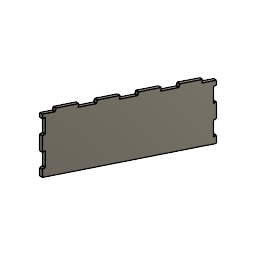
Deksel Volledig (Autodesk Fusion 360 archive; units mm, degrees)
design "de korte muur"
part number: 2026-02-05-13-28-29-515
part number: 2026-02-05-14-14-12-831
Autodesk Fusion 360 part; units mm, degrees
sketch "Sketch1" plane through (0, 0, 0) normal (0, 0, 1) x (1, 0, 0)
  line L0 (-114.5247, 50) -> (865.4753, 50)
  line L1 (865.4753, 50) -> (865.4753, -330)
  line L2 (865.4753, -330) -> (-114.5247, -330)
  line L3 (-114.5247, -330) -> (-114.5247, 50)
  line L4 (130.4753, 50) -> (130.4753, -330) construction
  line L5 (375.4753, -330) -> (375.4753, 50) construction
  line L6 (620.4753, 50) -> (620.4753, -330) construction
  line L7 (-39.5247, 0) -> (55.4753, 0)
  line L8 (80.4753, -25) -> (80.4753, -255)
  line L9 (55.4753, -280) -> (-39.5247, -280)
  line L10 (-64.5247, -255) -> (-64.5247, -25)
  line L11 (695.4753, 0) -> (790.4753, 0)
  line L12 (815.4753, -25) -> (815.4753, -255)
  line L13 (790.4753, -280) -> (695.4753, -280)
  line L14 (670.4753, -255) -> (670.4753, -25)
  arc A0 (-39.5247, 0) -> (-64.5247, -25) centre (-39.5247, -25) ccw
  arc A1 (80.4753, -25) -> (55.4753, 0) centre (55.4753, -25) ccw
  arc A2 (55.4753, -280) -> (80.4753, -255) centre (55.4753, -255) ccw
  arc A3 (-64.5247, -255) -> (-39.5247, -280) centre (-39.5247, -255) ccw
  arc A4 (670.4753, -255) -> (695.4753, -280) centre (695.4753, -255) ccw
  arc A5 (790.4753, -280) -> (815.4753, -255) centre (790.4753, -255) ccw
  arc A6 (695.4753, 0) -> (670.4753, -25) centre (695.4753, -25) ccw
  arc A7 (815.4753, -25) -> (790.4753, 0) centre (790.4753, -25) ccw
  line L15 (39.6391, 0) -> (711.3967, 0) construction
  line L16 (695.4753, -280) -> (677.7977, -280)
  line L17 (677.7977, -280) -> (25.0357, -280) construction
  line L18 (235.4753, -280) -> (270.4753, -280)
  line L19 (295.4753, -255) -> (295.4753, -25)
  line L20 (270.4753, 0) -> (235.4753, 0)
  line L21 (210.4753, -25) -> (210.4753, -255)
  arc A8 (210.4753, -255) -> (235.4753, -280) centre (235.4753, -255) ccw
  arc A9 (270.4753, -280) -> (295.4753, -255) centre (270.4753, -255) ccw
  arc A10 (235.4753, 0) -> (210.4753, -25) centre (235.4753, -25) ccw
  arc A11 (295.4753, -25) -> (270.4753, 0) centre (270.4753, -25) ccw
  line L22 (480.4753, 0) -> (515.4753, 0)
  line L23 (540.4753, -25) -> (540.4753, -255)
  line L24 (515.4753, -280) -> (480.4753, -280)
  line L25 (455.4753, -255) -> (455.4753, -25)
  arc A12 (455.4753, -255) -> (480.4753, -280) centre (480.4753, -255) ccw
  arc A13 (515.4753, -280) -> (540.4753, -255) centre (515.4753, -255) ccw
  arc A14 (540.4753, -25) -> (515.4753, 0) centre (515.4753, -25) ccw
  arc A15 (480.4753, 0) -> (455.4753, -25) centre (480.4753, -25) ccw
  line L26 (398.5325, -280) -> (398.5325, -272.6777)
  line L27 (497.9753, 0) -> (497.9753, -280) construction
  line L28 (455.4753, -140) -> (540.4753, -140) construction
  circle A16 centre (497.9753, -140) radius 75.0706
  dimension "d1" = 980
  dimension "d2" = 380
  dimension "d3" = 245
  dimension "d4" = 245
  dimension "d5" = 245
  dimension "d6" = 25
  dimension "d7" = 25
  dimension "d8" = 25
  dimension "d9" = 25
  dimension "d10" = 25
  dimension "d11" = 25
  dimension "d12" = 25
  dimension "d13" = 25
  dimension "d14" = 50
  dimension "d15" = 50
  dimension "d16" = 50
  dimension "d17" = 50
  dimension "d18" = 50
  dimension "d19" = 50
  dimension "d20" = 50
  dimension "d21" = 50
  dimension "d22" = 80
  dimension "d23" = 80
  dimension "d24" = 25
  dimension "d25" = 25
  dimension "d26" = 25
  dimension "d27" = 25
  dimension "d28" = 80
  dimension "d29" = 80
  dimension "d30" = 25
  dimension "d31" = 25
  dimension "d32" = 25
  dimension "d33" = 25
  constraint horizontal L0
  constraint vertical L1
  constraint horizontal L2
  constraint vertical L3
  constraint coincident L0 L4.start
  constraint coincident L2 L4.end
  constraint perpendicular L2 L4
  constraint coincident L2 L5.start
  constraint coincident L0 L5.end
  constraint perpendicular L0 L5
  constraint coincident L0 L6.start
  constraint coincident L2 L6.end
  constraint perpendicular L2 L6
  constraint horizontal L7
  constraint vertical L8
  constraint horizontal L9
  constraint vertical L10
  constraint horizontal L11
  constraint vertical L12
  constraint horizontal L13
  constraint vertical L14
  constraint tangent L7 A0
  constraint tangent L10 A0
  constraint tangent L7 A1
  constraint tangent L8 A1
  constraint tangent L8 A2
  constraint tangent L9 A2
  constraint tangent L9 A3
  constraint tangent L10 A3
  constraint tangent L13 A4
  constraint tangent L14 A4
  constraint tangent L12 A5
  constraint tangent L13 A5
  constraint tangent L11 A6
  constraint tangent L14 A6
  constraint tangent L11 A7
  constraint tangent L12 A7
  constraint coincident L7 L15.start
  constraint coincident L11 L15.end
  constraint tangent A4 L16
  constraint coincident L9 L17.end
  constraint horizontal L18
  constraint vertical L19
  constraint horizontal L20
  constraint vertical L21
  constraint tangent L18 A8
  constraint tangent L21 A8
  constraint tangent L18 A9
  constraint tangent L19 A9
  constraint tangent L20 A10
  constraint tangent L21 A10
  constraint tangent L19 A11
  constraint tangent L20 A11
  constraint horizontal L22
  constraint vertical L23
  constraint horizontal L24
  constraint vertical L25
  constraint tangent L24 A12
  constraint tangent L25 A12
  constraint tangent L23 A13
  constraint tangent L24 A13
  constraint tangent L22 A14
  constraint tangent L23 A14
  constraint tangent L22 A15
  constraint tangent L25 A15
  constraint coincident L17 L26.start
  constraint perpendicular L17 L26
  constraint midpoint L22 L27.start
  constraint midpoint L24 L27.end
  constraint midpoint L25 L28.start
  constraint midpoint L23 L28.end
  constraint midpoint L27 A16.centre
  measures "d1" distance of L0.start L0.end
  measures "d2" distance of L0.start L2.end
  measures "d3" distance of L3 L4
  measures "d4" distance of L4 L5
  measures "d5" distance of L5 L6
  measures "d6" radius of A0
  measures "d7" radius of A1
  measures "d8" radius of A2
  measures "d9" radius of A3
  measures "d10" radius of A4
  measures "d11" radius of A5
  measures "d12" radius of A6
  measures "d13" radius of A7
  measures "d14" distance of L3 L10
  measures "d15" distance of L0 L7
  measures "d16" distance of L4 L8
  measures "d17" distance of L2 L9
  measures "d18" distance of L2 L13
  measures "d19" distance of L1 L12
  measures "d20" distance of L6 L14
  measures "d21" distance of L0 L11
  measures "d22" distance of L4 L21
  measures "d23" distance of L5 L19
  measures "d24" radius of A8
  measures "d25" radius of A9
  measures "d26" radius of A10
  measures "d27" radius of A11
  measures "d28" distance of L5 L25
  measures "d29" distance of L6 L23
  measures "d30" radius of A12
  measures "d31" radius of A13
  measures "d32" radius of A14
  measures "d33" radius of A15
extrude "Extrude1" add sketch "Sketch1" along normal blind 6 makes body 1
sketch "Sketch2" plane through (0, 0, 6) normal (0, 0, 1) x (-1, 0, 0)
  arc A0 (-295.4753, 25) -> (-270.4753, 0) centre (-270.4753, 25) ccw
  line L0 (-295.4753, 25) -> (-295.4753, 255)
  arc A1 (-270.4753, 280) -> (-295.4753, 255) centre (-270.4753, 255) ccw
  line L1 (-270.4753, 280) -> (-235.4753, 280)
  arc A2 (-210.4753, 255) -> (-235.4753, 280) centre (-235.4753, 255) ccw
  line L2 (-210.4753, 255) -> (-210.4753, 25)
  arc A3 (-235.4753, 0) -> (-210.4753, 25) centre (-235.4753, 25) ccw
  line L3 (-235.4753, 0) -> (-270.4753, 0)
  arc A4 (39.5247, 0) -> (64.5247, 25) centre (39.5247, 25) ccw
  line L4 (39.5247, 0) -> (-55.4753, 0)
  arc A5 (-80.4753, 25) -> (-55.4753, 0) centre (-55.4753, 25) ccw
  line L5 (-80.4753, 25) -> (-80.4753, 255)
  arc A6 (-55.4753, 280) -> (-80.4753, 255) centre (-55.4753, 255) ccw
  line L6 (-55.4753, 280) -> (39.5247, 280)
  arc A7 (64.5247, 255) -> (39.5247, 280) centre (39.5247, 255) ccw
  line L7 (64.5247, 255) -> (64.5247, 25)
  arc A8 (-515.4753, 280) -> (-540.4753, 255) centre (-515.4753, 255) ccw
  line L8 (-515.4753, 280) -> (-480.4753, 280)
  arc A9 (-455.4753, 255) -> (-480.4753, 280) centre (-480.4753, 255) ccw
  line L9 (-455.4753, 255) -> (-455.4753, 201.8817)
  arc A10 (-455.4753, 78.1183) -> (-455.4753, 201.8817) centre (-497.9753, 140) ccw
  line L10 (-455.4753, 78.1183) -> (-455.4753, 25)
  arc A11 (-480.4753, 0) -> (-455.4753, 25) centre (-480.4753, 25) ccw
  line L11 (-480.4753, 0) -> (-515.4753, 0)
  arc A12 (-540.4753, 25) -> (-515.4753, 0) centre (-515.4753, 25) ccw
  line L12 (-540.4753, 25) -> (-540.4753, 78.1183)
  arc A13 (-540.4753, 201.8817) -> (-540.4753, 78.1183) centre (-497.9753, 140) ccw
  line L13 (-540.4753, 201.8817) -> (-540.4753, 255)
  arc A14 (-790.4753, 280) -> (-815.4753, 255) centre (-790.4753, 255) ccw
  line L14 (-790.4753, 280) -> (-695.4753, 280)
  arc A15 (-670.4753, 255) -> (-695.4753, 280) centre (-695.4753, 255) ccw
  line L15 (-670.4753, 255) -> (-670.4753, 25)
  arc A16 (-695.4753, 0) -> (-670.4753, 25) centre (-695.4753, 25) ccw
  line L16 (-695.4753, 0) -> (-790.4753, 0)
  arc A17 (-815.4753, 25) -> (-790.4753, 0) centre (-790.4753, 25) ccw
  line L17 (-815.4753, 25) -> (-815.4753, 255)
  line L18 (114.5247, 330) -> (-865.4753, 330)
  line L19 (-865.4753, 330) -> (-865.4753, -50)
  line L20 (-865.4753, -50) -> (114.5247, -50)
  line L21 (114.5247, -50) -> (114.5247, 330)
  line L22 (114.5247, 324) -> (-865.4753, 324) construction
  line L23 (108.5247, 330) -> (108.5247, -50) construction
  line L24 (114.5247, -44) -> (-865.4753, -44) construction
  line L25 (-859.4753, 330) -> (-859.4753, -50) construction
  line L26 (84.5247, 324) -> (84.5247, 330) construction
  line L27 (-835.4753, 324) -> (-835.4753, 330)
  line L28 (84.5247, 324) -> (34.5247, 324)
  line L29 (34.5247, 324) -> (34.5247, 330)
  line L30 (34.5247, 330) -> (84.5247, 330)
  line L31 (84.5247, 330) -> (84.5247, 324)
  line L32 (-12.142, 330) -> (-12.142, 324)
  line L33 (-62.142, 330) -> (-12.142, 330)
  line L34 (-12.142, 324) -> (-62.142, 324)
  line L35 (-62.142, 324) -> (-62.142, 330)
  line L36 (-108.8087, 330) -> (-108.8087, 324)
  line L37 (-158.8087, 330) -> (-108.8087, 330)
  line L38 (-108.8087, 324) -> (-158.8087, 324)
  line L39 (-158.8087, 324) -> (-158.8087, 330)
  line L40 (-205.4753, 330) -> (-205.4753, 324)
  line L41 (-255.4753, 330) -> (-205.4753, 330)
  line L42 (-205.4753, 324) -> (-255.4753, 324)
  line L43 (-255.4753, 324) -> (-255.4753, 330)
  line L44 (-302.142, 330) -> (-302.142, 324)
  line L45 (-352.142, 330) -> (-302.142, 330)
  line L46 (-302.142, 324) -> (-352.142, 324)
  line L47 (-352.142, 324) -> (-352.142, 330)
  line L48 (-398.8087, 330) -> (-398.8087, 324)
  line L49 (-448.8087, 330) -> (-398.8087, 330)
  line L50 (-398.8087, 324) -> (-448.8087, 324)
  line L51 (-448.8087, 324) -> (-448.8087, 330)
  line L52 (-495.4753, 330) -> (-495.4753, 324)
  line L53 (-545.4753, 330) -> (-495.4753, 330)
  line L54 (-495.4753, 324) -> (-545.4753, 324)
  line L55 (-545.4753, 324) -> (-545.4753, 330)
  line L56 (-592.142, 330) -> (-592.142, 324)
  line L57 (-642.142, 330) -> (-592.142, 330)
  line L58 (-592.142, 324) -> (-642.142, 324)
  line L59 (-642.142, 324) -> (-642.142, 330)
  line L60 (-688.8087, 330) -> (-688.8087, 324)
  line L61 (-738.8087, 330) -> (-688.8087, 330)
  line L62 (-688.8087, 324) -> (-738.8087, 324)
  line L63 (-738.8087, 324) -> (-738.8087, 330)
  line L64 (-785.4753, 330) -> (-785.4753, 324)
  line L65 (-835.4753, 330) -> (-785.4753, 330)
  line L66 (-785.4753, 324) -> (-835.4753, 324)
  line L67 (-835.4753, 324) -> (-835.4753, 330)
  line L68 (84.5247, 330) -> (84.5247, -212.2179) construction
  line L69 (-835.4753, 330) -> (-835.4753, -282.5126) construction
  line L70 (84.5247, -44) -> (34.5247, -44)
  line L71 (34.5247, -44) -> (34.5247, -50)
  line L72 (34.5247, -50) -> (84.5247, -50)
  line L73 (84.5247, -50) -> (84.5247, -44)
  line L74 (-12.142, -44) -> (-62.142, -44)
  line L75 (-12.142, -50) -> (-12.142, -44)
  line L76 (-62.142, -50) -> (-12.142, -50)
  line L77 (-62.142, -44) -> (-62.142, -50)
  line L78 (-108.8087, -44) -> (-158.8087, -44)
  line L79 (-108.8087, -50) -> (-108.8087, -44)
  line L80 (-158.8087, -50) -> (-108.8087, -50)
  line L81 (-158.8087, -44) -> (-158.8087, -50)
  line L82 (-205.4753, -44) -> (-255.4753, -44)
  line L83 (-205.4753, -50) -> (-205.4753, -44)
  line L84 (-255.4753, -50) -> (-205.4753, -50)
  line L85 (-255.4753, -44) -> (-255.4753, -50)
  line L86 (-302.142, -44) -> (-352.142, -44)
  line L87 (-302.142, -50) -> (-302.142, -44)
  line L88 (-352.142, -50) -> (-302.142, -50)
  line L89 (-352.142, -44) -> (-352.142, -50)
  line L90 (-398.8087, -44) -> (-448.8087, -44)
  line L91 (-398.8087, -50) -> (-398.8087, -44)
  line L92 (-448.8087, -50) -> (-398.8087, -50)
  line L93 (-448.8087, -44) -> (-448.8087, -50)
  line L94 (-495.4753, -44) -> (-545.4753, -44)
  line L95 (-495.4753, -50) -> (-495.4753, -44)
  line L96 (-545.4753, -50) -> (-495.4753, -50)
  line L97 (-545.4753, -44) -> (-545.4753, -50)
  line L98 (-592.142, -44) -> (-642.142, -44)
  line L99 (-592.142, -50) -> (-592.142, -44)
  line L100 (-642.142, -50) -> (-592.142, -50)
  line L101 (-642.142, -44) -> (-642.142, -50)
  line L102 (-688.8087, -44) -> (-738.8087, -44)
  line L103 (-688.8087, -50) -> (-688.8087, -44)
  line L104 (-738.8087, -50) -> (-688.8087, -50)
  line L105 (-738.8087, -44) -> (-738.8087, -50)
  line L106 (-785.4753, -44) -> (-835.4753, -44)
  line L107 (-785.4753, -50) -> (-785.4753, -44)
  line L108 (-835.4753, -50) -> (-785.4753, -50)
  line L109 (-835.4753, -44) -> (-835.4753, -50)
  line L110 (128.1385, 300) -> (-1003.4541, 300) construction
  line L111 (150.6287, -20) -> (-1059.1196, -20) construction
  line L112 (108.5247, 300) -> (114.5247, 300)
  line L113 (114.5247, 300) -> (114.5247, 250)
  line L114 (114.5247, 250) -> (108.5247, 250)
  line L115 (108.5247, 250) -> (108.5247, 300)
  line L116 (114.5247, 210) -> (114.5247, 160)
  line L117 (114.5247, 160) -> (108.5247, 160)
  line L118 (108.5247, 160) -> (108.5247, 210)
  line L119 (108.5247, 210) -> (114.5247, 210)
  line L120 (114.5247, 120) -> (114.5247, 70)
  line L121 (114.5247, 70) -> (108.5247, 70)
  line L122 (108.5247, 70) -> (108.5247, 120)
  line L123 (108.5247, 120) -> (114.5247, 120)
  line L124 (114.5247, 30) -> (114.5247, -20)
  line L125 (114.5247, -20) -> (108.5247, -20)
  line L126 (108.5247, -20) -> (108.5247, 30)
  line L127 (108.5247, 30) -> (114.5247, 30)
  line L128 (-865.4753, 300) -> (-859.4753, 300)
  line L129 (-859.4753, 300) -> (-859.4753, 250)
  line L130 (-859.4753, 250) -> (-865.4753, 250)
  line L131 (-865.4753, 250) -> (-865.4753, 300)
  line L132 (-865.4753, 210) -> (-859.4753, 210)
  line L133 (-859.4753, 210) -> (-859.4753, 160)
  line L134 (-865.4753, 160) -> (-865.4753, 210)
  line L135 (-859.4753, 160) -> (-865.4753, 160)
  line L136 (-865.4753, 120) -> (-859.4753, 120)
  line L137 (-859.4753, 120) -> (-859.4753, 70)
  line L138 (-865.4753, 70) -> (-865.4753, 120)
  line L139 (-859.4753, 70) -> (-865.4753, 70)
  line L140 (-865.4753, 30) -> (-859.4753, 30)
  line L141 (-859.4753, 30) -> (-859.4753, -20)
  line L142 (-865.4753, -20) -> (-865.4753, 30)
  line L143 (-859.4753, -20) -> (-865.4753, -20)
  dimension "d37" = 6
  dimension "d38" = 6
  dimension "d39" = 6
  dimension "d40" = 6
  dimension "d42" = 30
  dimension "d43" = 30
  dimension "d44" = 50
  dimension "d47" = -870
  dimension "d48" = 0
  dimension "d49" = 50
  dimension "d52" = -870
  dimension "d53" = 0
  dimension "d54" = 30
  dimension "d55" = 30
  dimension "d56" = 50
  dimension "d59" = 0
  dimension "d60" = -270
  dimension "d61" = 50
  dimension "d64" = 0
  dimension "d65" = -270
  constraint coincident L21 L22.start
  constraint coincident L19 L22.end
  constraint perpendicular L19 L22
  constraint coincident L18 L23.start
  constraint coincident L20 L23.end
  constraint perpendicular L20 L23
  constraint coincident L21 L24.start
  constraint coincident L19 L24.end
  constraint perpendicular L19 L24
  constraint coincident L18 L25.start
  constraint coincident L20 L25.end
  constraint perpendicular L20 L25
  constraint coincident L22 L26.start
  constraint coincident L18 L26.end
  constraint perpendicular L18 L26
  constraint coincident L22 L27.start
  constraint coincident L18 L27.end
  constraint perpendicular L18 L27
  constraint horizontal L28
  constraint vertical L29
  constraint horizontal L30
  constraint vertical L31
  constraint coincident L18 L29.end
  constraint perpendicular L28 L68
  constraint perpendicular L20 L69
  constraint horizontal L70
  constraint vertical L71
  constraint horizontal L72
  constraint vertical L73
  constraint coincident L20 L71.end
  constraint coincident L68 L70.start
  constraint coincident L24 L70.start
  constraint perpendicular L25 L110
  constraint perpendicular L103 L111
  constraint horizontal L112
  constraint vertical L113
  constraint horizontal L114
  constraint vertical L115
  constraint coincident L21 L113.end
  constraint coincident L110 L112.start
  constraint coincident L23 L112.start
  constraint horizontal L128
  constraint vertical L129
  constraint horizontal L130
  constraint vertical L131
  constraint coincident L25 L129.end
  constraint coincident L19 L128.start
  constraint coincident L110 L128.start
  measures "d37" distance of L21 L23
  measures "d38" distance of L20 L24
  measures "d39" distance of L19 L25
  measures "d40" distance of L18 L22
  measures "d42" distance of L21 L26
  measures "d43" distance of L19 L27
  measures "d44" distance of L26.start L28.end
  measures "d49" distance of L70.start L70.end
  measures "d54" distance of L20 L111
  measures "d55" distance of L18 L110
  measures "d56" distance of L112.start L114.end
  measures "d61" distance of L128.start L130.end
extrude "Extrude2" cut sketch "Sketch2" against normal blind 40 contours L18 L28 L29 L30 L31 | L21 L112 L113 L114 L115 | L18 L32 L33 L34 L35 | L21 L116 L117 L118 L119 | L18 L36 L37 L38 L39 | L21 L120 L121 L122 L123 | L18 L40 L41 L42 L43 | L21 L124 L125 L126 L127 | L18 L44 L45 L46 L47 | L20 L70 L71 L72 L73 | L18 L48 L49 L50 L51 | L20 L74 L75 L76 L77 | L18 L52 L53 L54 L55 | L20 L78 L79 L80 L81 | L18 L56 L57 L58 L59 | L20 L82 L83 L84 L85 | L18 L60 L61 L62 L63 | L20 L86 L87 L88 L89 | L18 L27 L64 L65 L66 L67 | L20 L90 L91 L92 L93 | L19 L128 L129 L130 L131 | L20 L94 L95 L96 L97 | L19 L132 L133 L134 L135 | L20 L98 L99 L100 L101 | L19 L136 L137 L138 L139 | L20 L102 L103 L104 L105 | L19 L140 L141 L142 L143 | L20 L106 L107 L108 L109 bodies 1
move_body "Move1" bodies 1 to x (1, 0, 0) y (0, 0.949425, -0.313992) z (0, 0.313992, 0.949425) at (0, -16.6896, 196.3825)
sketch "Sketch1 (2)" plane through (-114.5247, 0, 0) normal (-1, 0, 0) x (0, -1, 0) in component "Component"
  line L0 (299.6333, 296.2768) -> (301.5172, 290.5802)
  line L1 (301.5172, 290.5802) -> (330, 300)
  line L2 (330, 300) -> (328.116, 305.6966)
  line L3 (328.116, 305.6966) -> (299.6333, 296.2768)
  line L4 (299.6333, 296.2768) -> (328.116, 305.6966)
  line L5 (-32.6656, 186.3794) -> (-4.1829, 195.7992)
  line L6 (-32.6656, 186.3794) -> (-32.6656, 66.3794)
  line L7 (-32.6656, 186.3794) -> (328.116, 305.6966)
  line L8 (328.116, 305.6966) -> (328.116, 185.6966)
  line L9 (-32.6656, 66.3794) -> (328.116, 185.6966)
  line L10 (-32.6656, 81.3794) -> (-26.6656, 81.3794)
  line L11 (-26.6656, 81.3794) -> (-26.6656, 111.3794)
  line L12 (-26.6656, 111.3794) -> (-32.6656, 111.3794)
  line L13 (-32.6656, 111.3794) -> (-32.6656, 81.3794)
  line L14 (-32.6656, 141.3794) -> (-26.6656, 141.3794)
  line L15 (-26.6656, 141.3794) -> (-26.6656, 171.3794)
  line L16 (-26.6656, 171.3794) -> (-32.6656, 171.3794)
  line L17 (-32.6656, 171.3794) -> (-32.6656, 141.3794)
  line L18 (328.116, 200.6966) -> (322.116, 200.6966)
  line L19 (322.116, 200.6966) -> (322.116, 230.6966)
  line L20 (322.116, 230.6966) -> (328.116, 230.6966)
  line L21 (328.116, 230.6966) -> (328.116, 200.6966)
  line L22 (328.116, 260.6966) -> (322.116, 260.6966)
  line L23 (322.116, 260.6966) -> (322.116, 290.6966)
  line L24 (322.116, 290.6966) -> (328.116, 290.6966)
  line L25 (328.116, 290.6966) -> (328.116, 260.6966)
  dimension "d68" = 120
  dimension "d69" = 120
  dimension "d70" = 6
  dimension "d71" = 30
  dimension "d72" = 30
  dimension "d73" = 6
  dimension "d74" = 30
  dimension "d75" = 6
  dimension "d76" = 30
  dimension "d77" = 6
  dimension "d82" = 30
  dimension "d83" = 30
  dimension "d84" = 15
  dimension "d85" = 15
  constraint coincident L5.start L6.start
  constraint vertical L6
  constraint coincident L2.end L3.start
  constraint vertical L8
  constraint horizontal L10
  constraint vertical L11
  constraint horizontal L12
  constraint vertical L13
  constraint coincident L6 L10.start
  constraint horizontal L14
  constraint vertical L15
  constraint horizontal L16
  constraint vertical L17
  constraint coincident L6 L14.start
  constraint horizontal L18
  constraint vertical L19
  constraint horizontal L20
  constraint vertical L21
  constraint coincident L8 L18.start
  constraint horizontal L22
  constraint vertical L23
  constraint horizontal L24
  constraint vertical L25
  constraint coincident L8 L22.start
  measures "d68" distance of L5.start L6.end
  measures "d69" distance of L2.end L8.end
  measures "d70" distance of L10.start L10.end
  measures "d71" distance of L10.end L11.end
  measures "d72" distance of L14.start L16.end
  measures "d73" distance of L14.start L14.end
  measures "d74" distance of L18.start L20.end
  measures "d75" distance of L19.end L20.end
  measures "d76" distance of L22.start L24.end
  measures "d77" distance of L22.start L22.end
  measures "d82" distance of L20 L22
  measures "d83" distance of L12 L14
  measures "d84" distance of L6.end L10.start
  measures "d85" distance of L8.end L18.start
extrude "Extrude1'" add sketch "Sketch1 (2)" against normal blind 6 separate body contours L0 L1 L5 L6 L7 L8 L9 L10 L11 L12 L14 L15 L16 L18 L19 L20 L22 L23 L24 makes body 2 in component "Component"
combine "Combine1" operation cut target body 2 tool bodies 1 in component "Component"
sketch "Sketch2 (2)" plane through (-114.5247, 0, 0) normal (-1, 0, 0) x (0, -1, 0) in component "Component"
  line L0 (-30.7817, 180.6829) -> (-32.6656, 186.3794)
  line L1 (-32.6656, 186.3794) -> (-32.6656, 171.3794)
  line L2 (-32.6656, 171.3794) -> (-26.6656, 171.3794)
  line L3 (-26.6656, 171.3794) -> (-26.6656, 141.3794)
  line L4 (-26.6656, 141.3794) -> (-32.6656, 141.3794)
  line L5 (-32.6656, 141.3794) -> (-32.6656, 111.3794)
  line L6 (-32.6656, 111.3794) -> (-26.6656, 111.3794)
  line L7 (-26.6656, 111.3794) -> (-26.6656, 81.3794)
  line L8 (-26.6656, 81.3794) -> (-32.6656, 81.3794)
  line L9 (-32.6656, 81.3794) -> (-32.6656, 66.3794)
  line L10 (-32.6656, 66.3794) -> (328.116, 185.6966)
  line L11 (328.116, 185.6966) -> (328.116, 200.6966)
  line L12 (328.116, 200.6966) -> (322.116, 200.6966)
  line L13 (322.116, 200.6966) -> (322.116, 230.6966)
  line L14 (322.116, 230.6966) -> (328.116, 230.6966)
  line L15 (328.116, 230.6966) -> (328.116, 260.6966)
  line L16 (328.116, 260.6966) -> (322.116, 260.6966)
  line L17 (322.116, 260.6966) -> (322.116, 290.6966)
  line L18 (322.116, 290.6966) -> (328.116, 290.6966)
  line L19 (328.116, 290.6966) -> (328.116, 299.3769)
  line L20 (328.116, 299.3769) -> (301.5172, 290.5802)
  line L21 (301.5172, 290.5802) -> (299.6333, 296.2768)
  line L22 (299.6333, 296.2768) -> (252.162, 280.5772)
  line L23 (252.162, 280.5772) -> (254.046, 274.8806)
  line L24 (254.046, 274.8806) -> (216.0689, 262.3209)
  line L25 (216.0689, 262.3209) -> (214.185, 268.0175)
  line L26 (214.185, 268.0175) -> (166.7137, 252.3178)
  line L27 (166.7137, 252.3178) -> (168.5977, 246.6213)
  line L28 (168.5977, 246.6213) -> (130.6206, 234.0616)
  line L29 (130.6206, 234.0616) -> (128.7367, 239.7581)
  line L30 (128.7367, 239.7581) -> (81.2654, 224.0585)
  line L31 (81.2654, 224.0585) -> (83.1494, 218.362)
  line L32 (83.1494, 218.362) -> (45.1724, 205.8023)
  line L33 (45.1724, 205.8023) -> (43.2884, 211.4988)
  line L34 (43.2884, 211.4988) -> (-4.1829, 195.7992)
  line L35 (-4.1829, 195.7992) -> (-2.2989, 190.1026)
  line L36 (-2.2989, 190.1026) -> (-30.7817, 180.6829)
  line L37 (-30.7817, 180.6829) -> (-32.6656, 180.0598)
  constraint coincident L0.start L36.end
  constraint coincident L1 L37.end
  constraint perpendicular L0 L37
extrude "Extrude2'" cut sketch "Sketch2 (2)" against normal blind 19 contours L0 L1 L37 bodies 2 in component "Component"
component "Component" placed x (1, 0, 0) y (0, 1, 0) z (0, 0, 1) at (0, 0, 0)
equation "d7 = d6"
equation "d8 = d6"
equation "d10 = d6"
equation "d12 = d6"
equation "d23 = d22"
equation "d24 = d6"
equation "d28 = d22"
equation "d29 = d22"
equation "d30 = d6"
equation "d31 = d6"
equation "d32 = d6"
equation "d33 = d6"

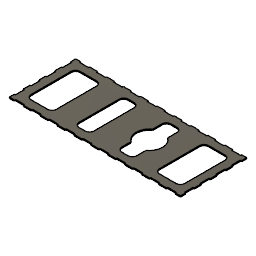
design "muur kort"
part number: 2026-02-05-13-28-29-515
Autodesk Fusion 360 part; units mm, degrees
sketch "Sketch1" plane through (0, 0, 0) normal (0, 0, 1) x (1, 0, 0)
  line L0 (-114.5247, 50) -> (865.4753, 50)
  line L1 (865.4753, 50) -> (865.4753, -330)
  line L2 (865.4753, -330) -> (-114.5247, -330)
  line L3 (-114.5247, -330) -> (-114.5247, 50)
  line L4 (130.4753, 50) -> (130.4753, -330) construction
  line L5 (375.4753, -330) -> (375.4753, 50) construction
  line L6 (620.4753, 50) -> (620.4753, -330) construction
  line L7 (-39.5247, 0) -> (55.4753, 0)
  line L8 (80.4753, -25) -> (80.4753, -255)
  line L9 (55.4753, -280) -> (-39.5247, -280)
  line L10 (-64.5247, -255) -> (-64.5247, -25)
  line L11 (695.4753, 0) -> (790.4753, 0)
  line L12 (815.4753, -25) -> (815.4753, -255)
  line L13 (790.4753, -280) -> (695.4753, -280)
  line L14 (670.4753, -255) -> (670.4753, -25)
  arc A0 (-39.5247, 0) -> (-64.5247, -25) centre (-39.5247, -25) ccw
  arc A1 (80.4753, -25) -> (55.4753, 0) centre (55.4753, -25) ccw
  arc A2 (55.4753, -280) -> (80.4753, -255) centre (55.4753, -255) ccw
  arc A3 (-64.5247, -255) -> (-39.5247, -280) centre (-39.5247, -255) ccw
  arc A4 (670.4753, -255) -> (695.4753, -280) centre (695.4753, -255) ccw
  arc A5 (790.4753, -280) -> (815.4753, -255) centre (790.4753, -255) ccw
  arc A6 (695.4753, 0) -> (670.4753, -25) centre (695.4753, -25) ccw
  arc A7 (815.4753, -25) -> (790.4753, 0) centre (790.4753, -25) ccw
  line L15 (39.6391, 0) -> (711.3967, 0) construction
  line L16 (695.4753, -280) -> (677.7977, -280)
  line L17 (677.7977, -280) -> (25.0357, -280) construction
  line L18 (235.4753, -280) -> (270.4753, -280)
  line L19 (295.4753, -255) -> (295.4753, -25)
  line L20 (270.4753, 0) -> (235.4753, 0)
  line L21 (210.4753, -25) -> (210.4753, -255)
  arc A8 (210.4753, -255) -> (235.4753, -280) centre (235.4753, -255) ccw
  arc A9 (270.4753, -280) -> (295.4753, -255) centre (270.4753, -255) ccw
  arc A10 (235.4753, 0) -> (210.4753, -25) centre (235.4753, -25) ccw
  arc A11 (295.4753, -25) -> (270.4753, 0) centre (270.4753, -25) ccw
  line L22 (480.4753, 0) -> (515.4753, 0)
  line L23 (540.4753, -25) -> (540.4753, -255)
  line L24 (515.4753, -280) -> (480.4753, -280)
  line L25 (455.4753, -255) -> (455.4753, -25)
  arc A12 (455.4753, -255) -> (480.4753, -280) centre (480.4753, -255) ccw
  arc A13 (515.4753, -280) -> (540.4753, -255) centre (515.4753, -255) ccw
  arc A14 (540.4753, -25) -> (515.4753, 0) centre (515.4753, -25) ccw
  arc A15 (480.4753, 0) -> (455.4753, -25) centre (480.4753, -25) ccw
  line L26 (398.5325, -280) -> (398.5325, -272.6777)
  line L27 (497.9753, 0) -> (497.9753, -280) construction
  line L28 (455.4753, -140) -> (540.4753, -140) construction
  circle A16 centre (497.9753, -140) radius 75.0706
  dimension "d1" = 980
  dimension "d2" = 380
  dimension "d3" = 245
  dimension "d4" = 245
  dimension "d5" = 245
  dimension "d6" = 25
  dimension "d7" = 25
  dimension "d8" = 25
  dimension "d9" = 25
  dimension "d10" = 25
  dimension "d11" = 25
  dimension "d12" = 25
  dimension "d13" = 25
  dimension "d14" = 50
  dimension "d15" = 50
  dimension "d16" = 50
  dimension "d17" = 50
  dimension "d18" = 50
  dimension "d19" = 50
  dimension "d20" = 50
  dimension "d21" = 50
  dimension "d22" = 80
  dimension "d23" = 80
  dimension "d24" = 25
  dimension "d25" = 25
  dimension "d26" = 25
  dimension "d27" = 25
  dimension "d28" = 80
  dimension "d29" = 80
  dimension "d30" = 25
  dimension "d31" = 25
  dimension "d32" = 25
  dimension "d33" = 25
  constraint horizontal L0
  constraint vertical L1
  constraint horizontal L2
  constraint vertical L3
  constraint coincident L0 L4.start
  constraint coincident L2 L4.end
  constraint perpendicular L2 L4
  constraint coincident L2 L5.start
  constraint coincident L0 L5.end
  constraint perpendicular L0 L5
  constraint coincident L0 L6.start
  constraint coincident L2 L6.end
  constraint perpendicular L2 L6
  constraint horizontal L7
  constraint vertical L8
  constraint horizontal L9
  constraint vertical L10
  constraint horizontal L11
  constraint vertical L12
  constraint horizontal L13
  constraint vertical L14
  constraint tangent L7 A0
  constraint tangent L10 A0
  constraint tangent L7 A1
  constraint tangent L8 A1
  constraint tangent L8 A2
  constraint tangent L9 A2
  constraint tangent L9 A3
  constraint tangent L10 A3
  constraint tangent L13 A4
  constraint tangent L14 A4
  constraint tangent L12 A5
  constraint tangent L13 A5
  constraint tangent L11 A6
  constraint tangent L14 A6
  constraint tangent L11 A7
  constraint tangent L12 A7
  constraint coincident L7 L15.start
  constraint coincident L11 L15.end
  constraint tangent A4 L16
  constraint coincident L9 L17.end
  constraint horizontal L18
  constraint vertical L19
  constraint horizontal L20
  constraint vertical L21
  constraint tangent L18 A8
  constraint tangent L21 A8
  constraint tangent L18 A9
  constraint tangent L19 A9
  constraint tangent L20 A10
  constraint tangent L21 A10
  constraint tangent L19 A11
  constraint tangent L20 A11
  constraint horizontal L22
  constraint vertical L23
  constraint horizontal L24
  constraint vertical L25
  constraint tangent L24 A12
  constraint tangent L25 A12
  constraint tangent L23 A13
  constraint tangent L24 A13
  constraint tangent L22 A14
  constraint tangent L23 A14
  constraint tangent L22 A15
  constraint tangent L25 A15
  constraint coincident L17 L26.start
  constraint perpendicular L17 L26
  constraint midpoint L22 L27.start
  constraint midpoint L24 L27.end
  constraint midpoint L25 L28.start
  constraint midpoint L23 L28.end
  constraint midpoint L27 A16.centre
  measures "d1" distance of L0.start L0.end
  measures "d2" distance of L0.start L2.end
  measures "d3" distance of L3 L4
  measures "d4" distance of L4 L5
  measures "d5" distance of L5 L6
  measures "d6" radius of A0
  measures "d7" radius of A1
  measures "d8" radius of A2
  measures "d9" radius of A3
  measures "d10" radius of A4
  measures "d11" radius of A5
  measures "d12" radius of A6
  measures "d13" radius of A7
  measures "d14" distance of L3 L10
  measures "d15" distance of L0 L7
  measures "d16" distance of L4 L8
  measures "d17" distance of L2 L9
  measures "d18" distance of L2 L13
  measures "d19" distance of L1 L12
  measures "d20" distance of L6 L14
  measures "d21" distance of L0 L11
  measures "d22" distance of L4 L21
  measures "d23" distance of L5 L19
  measures "d24" radius of A8
  measures "d25" radius of A9
  measures "d26" radius of A10
  measures "d27" radius of A11
  measures "d28" distance of L5 L25
  measures "d29" distance of L6 L23
  measures "d30" radius of A12
  measures "d31" radius of A13
  measures "d32" radius of A14
  measures "d33" radius of A15
extrude "Extrude1" add sketch "Sketch1" along normal blind 6
sketch "Sketch2" plane through (0, 0, 6) normal (0, 0, 1) x (-1, 0, 0)
  arc A0 (-295.4753, 25) -> (-270.4753, 0) centre (-270.4753, 25) ccw
  line L0 (-295.4753, 25) -> (-295.4753, 255)
  arc A1 (-270.4753, 280) -> (-295.4753, 255) centre (-270.4753, 255) ccw
  line L1 (-270.4753, 280) -> (-235.4753, 280)
  arc A2 (-210.4753, 255) -> (-235.4753, 280) centre (-235.4753, 255) ccw
  line L2 (-210.4753, 255) -> (-210.4753, 25)
  arc A3 (-235.4753, 0) -> (-210.4753, 25) centre (-235.4753, 25) ccw
  line L3 (-235.4753, 0) -> (-270.4753, 0)
  arc A4 (39.5247, 0) -> (64.5247, 25) centre (39.5247, 25) ccw
  line L4 (39.5247, 0) -> (-55.4753, 0)
  arc A5 (-80.4753, 25) -> (-55.4753, 0) centre (-55.4753, 25) ccw
  line L5 (-80.4753, 25) -> (-80.4753, 255)
  arc A6 (-55.4753, 280) -> (-80.4753, 255) centre (-55.4753, 255) ccw
  line L6 (-55.4753, 280) -> (39.5247, 280)
  arc A7 (64.5247, 255) -> (39.5247, 280) centre (39.5247, 255) ccw
  line L7 (64.5247, 255) -> (64.5247, 25)
  arc A8 (-515.4753, 280) -> (-540.4753, 255) centre (-515.4753, 255) ccw
  line L8 (-515.4753, 280) -> (-480.4753, 280)
  arc A9 (-455.4753, 255) -> (-480.4753, 280) centre (-480.4753, 255) ccw
  line L9 (-455.4753, 255) -> (-455.4753, 201.8817)
  arc A10 (-455.4753, 78.1183) -> (-455.4753, 201.8817) centre (-497.9753, 140) ccw
  line L10 (-455.4753, 78.1183) -> (-455.4753, 25)
  arc A11 (-480.4753, 0) -> (-455.4753, 25) centre (-480.4753, 25) ccw
  line L11 (-480.4753, 0) -> (-515.4753, 0)
  arc A12 (-540.4753, 25) -> (-515.4753, 0) centre (-515.4753, 25) ccw
  line L12 (-540.4753, 25) -> (-540.4753, 78.1183)
  arc A13 (-540.4753, 201.8817) -> (-540.4753, 78.1183) centre (-497.9753, 140) ccw
  line L13 (-540.4753, 201.8817) -> (-540.4753, 255)
  arc A14 (-790.4753, 280) -> (-815.4753, 255) centre (-790.4753, 255) ccw
  line L14 (-790.4753, 280) -> (-695.4753, 280)
  arc A15 (-670.4753, 255) -> (-695.4753, 280) centre (-695.4753, 255) ccw
  line L15 (-670.4753, 255) -> (-670.4753, 25)
  arc A16 (-695.4753, 0) -> (-670.4753, 25) centre (-695.4753, 25) ccw
  line L16 (-695.4753, 0) -> (-790.4753, 0)
  arc A17 (-815.4753, 25) -> (-790.4753, 0) centre (-790.4753, 25) ccw
  line L17 (-815.4753, 25) -> (-815.4753, 255)
  line L18 (114.5247, 330) -> (-865.4753, 330)
  line L19 (-865.4753, 330) -> (-865.4753, -50)
  line L20 (-865.4753, -50) -> (114.5247, -50)
  line L21 (114.5247, -50) -> (114.5247, 330)
  line L22 (114.5247, 324) -> (-865.4753, 324) construction
  line L23 (108.5247, 330) -> (108.5247, -50) construction
  line L24 (114.5247, -44) -> (-865.4753, -44) construction
  line L25 (-859.4753, 330) -> (-859.4753, -50) construction
  line L26 (84.5247, 324) -> (84.5247, 330) construction
  line L27 (-835.4753, 324) -> (-835.4753, 330)
  line L28 (84.5247, 324) -> (34.5247, 324)
  line L29 (34.5247, 324) -> (34.5247, 330)
  line L30 (34.5247, 330) -> (84.5247, 330)
  line L31 (84.5247, 330) -> (84.5247, 324)
  line L32 (-12.142, 330) -> (-12.142, 324)
  line L33 (-62.142, 330) -> (-12.142, 330)
  line L34 (-12.142, 324) -> (-62.142, 324)
  line L35 (-62.142, 324) -> (-62.142, 330)
  line L36 (-108.8087, 330) -> (-108.8087, 324)
  line L37 (-158.8087, 330) -> (-108.8087, 330)
  line L38 (-108.8087, 324) -> (-158.8087, 324)
  line L39 (-158.8087, 324) -> (-158.8087, 330)
  line L40 (-205.4753, 330) -> (-205.4753, 324)
  line L41 (-255.4753, 330) -> (-205.4753, 330)
  line L42 (-205.4753, 324) -> (-255.4753, 324)
  line L43 (-255.4753, 324) -> (-255.4753, 330)
  line L44 (-302.142, 330) -> (-302.142, 324)
  line L45 (-352.142, 330) -> (-302.142, 330)
  line L46 (-302.142, 324) -> (-352.142, 324)
  line L47 (-352.142, 324) -> (-352.142, 330)
  line L48 (-398.8087, 330) -> (-398.8087, 324)
  line L49 (-448.8087, 330) -> (-398.8087, 330)
  line L50 (-398.8087, 324) -> (-448.8087, 324)
  line L51 (-448.8087, 324) -> (-448.8087, 330)
  line L52 (-495.4753, 330) -> (-495.4753, 324)
  line L53 (-545.4753, 330) -> (-495.4753, 330)
  line L54 (-495.4753, 324) -> (-545.4753, 324)
  line L55 (-545.4753, 324) -> (-545.4753, 330)
  line L56 (-592.142, 330) -> (-592.142, 324)
  line L57 (-642.142, 330) -> (-592.142, 330)
  line L58 (-592.142, 324) -> (-642.142, 324)
  line L59 (-642.142, 324) -> (-642.142, 330)
  line L60 (-688.8087, 330) -> (-688.8087, 324)
  line L61 (-738.8087, 330) -> (-688.8087, 330)
  line L62 (-688.8087, 324) -> (-738.8087, 324)
  line L63 (-738.8087, 324) -> (-738.8087, 330)
  line L64 (-785.4753, 330) -> (-785.4753, 324)
  line L65 (-835.4753, 330) -> (-785.4753, 330)
  line L66 (-785.4753, 324) -> (-835.4753, 324)
  line L67 (-835.4753, 324) -> (-835.4753, 330)
  line L68 (84.5247, 330) -> (84.5247, -212.2179) construction
  line L69 (-835.4753, 330) -> (-835.4753, -282.5126) construction
  line L70 (84.5247, -44) -> (34.5247, -44)
  line L71 (34.5247, -44) -> (34.5247, -50)
  line L72 (34.5247, -50) -> (84.5247, -50)
  line L73 (84.5247, -50) -> (84.5247, -44)
  line L74 (-12.142, -44) -> (-62.142, -44)
  line L75 (-12.142, -50) -> (-12.142, -44)
  line L76 (-62.142, -50) -> (-12.142, -50)
  line L77 (-62.142, -44) -> (-62.142, -50)
  line L78 (-108.8087, -44) -> (-158.8087, -44)
  line L79 (-108.8087, -50) -> (-108.8087, -44)
  line L80 (-158.8087, -50) -> (-108.8087, -50)
  line L81 (-158.8087, -44) -> (-158.8087, -50)
  line L82 (-205.4753, -44) -> (-255.4753, -44)
  line L83 (-205.4753, -50) -> (-205.4753, -44)
  line L84 (-255.4753, -50) -> (-205.4753, -50)
  line L85 (-255.4753, -44) -> (-255.4753, -50)
  line L86 (-302.142, -44) -> (-352.142, -44)
  line L87 (-302.142, -50) -> (-302.142, -44)
  line L88 (-352.142, -50) -> (-302.142, -50)
  line L89 (-352.142, -44) -> (-352.142, -50)
  line L90 (-398.8087, -44) -> (-448.8087, -44)
  line L91 (-398.8087, -50) -> (-398.8087, -44)
  line L92 (-448.8087, -50) -> (-398.8087, -50)
  line L93 (-448.8087, -44) -> (-448.8087, -50)
  line L94 (-495.4753, -44) -> (-545.4753, -44)
  line L95 (-495.4753, -50) -> (-495.4753, -44)
  line L96 (-545.4753, -50) -> (-495.4753, -50)
  line L97 (-545.4753, -44) -> (-545.4753, -50)
  line L98 (-592.142, -44) -> (-642.142, -44)
  line L99 (-592.142, -50) -> (-592.142, -44)
  line L100 (-642.142, -50) -> (-592.142, -50)
  line L101 (-642.142, -44) -> (-642.142, -50)
  line L102 (-688.8087, -44) -> (-738.8087, -44)
  line L103 (-688.8087, -50) -> (-688.8087, -44)
  line L104 (-738.8087, -50) -> (-688.8087, -50)
  line L105 (-738.8087, -44) -> (-738.8087, -50)
  line L106 (-785.4753, -44) -> (-835.4753, -44)
  line L107 (-785.4753, -50) -> (-785.4753, -44)
  line L108 (-835.4753, -50) -> (-785.4753, -50)
  line L109 (-835.4753, -44) -> (-835.4753, -50)
  line L110 (128.1385, 300) -> (-1003.4541, 300) construction
  line L111 (150.6287, -20) -> (-1059.1196, -20) construction
  line L112 (108.5247, 300) -> (114.5247, 300)
  line L113 (114.5247, 300) -> (114.5247, 250)
  line L114 (114.5247, 250) -> (108.5247, 250)
  line L115 (108.5247, 250) -> (108.5247, 300)
  line L116 (114.5247, 210) -> (114.5247, 160)
  line L117 (114.5247, 160) -> (108.5247, 160)
  line L118 (108.5247, 160) -> (108.5247, 210)
  line L119 (108.5247, 210) -> (114.5247, 210)
  line L120 (114.5247, 120) -> (114.5247, 70)
  line L121 (114.5247, 70) -> (108.5247, 70)
  line L122 (108.5247, 70) -> (108.5247, 120)
  line L123 (108.5247, 120) -> (114.5247, 120)
  line L124 (114.5247, 30) -> (114.5247, -20)
  line L125 (114.5247, -20) -> (108.5247, -20)
  line L126 (108.5247, -20) -> (108.5247, 30)
  line L127 (108.5247, 30) -> (114.5247, 30)
  line L128 (-865.4753, 300) -> (-859.4753, 300)
  line L129 (-859.4753, 300) -> (-859.4753, 250)
  line L130 (-859.4753, 250) -> (-865.4753, 250)
  line L131 (-865.4753, 250) -> (-865.4753, 300)
  line L132 (-865.4753, 210) -> (-859.4753, 210)
  line L133 (-859.4753, 210) -> (-859.4753, 160)
  line L134 (-865.4753, 160) -> (-865.4753, 210)
  line L135 (-859.4753, 160) -> (-865.4753, 160)
  line L136 (-865.4753, 120) -> (-859.4753, 120)
  line L137 (-859.4753, 120) -> (-859.4753, 70)
  line L138 (-865.4753, 70) -> (-865.4753, 120)
  line L139 (-859.4753, 70) -> (-865.4753, 70)
  line L140 (-865.4753, 30) -> (-859.4753, 30)
  line L141 (-859.4753, 30) -> (-859.4753, -20)
  line L142 (-865.4753, -20) -> (-865.4753, 30)
  line L143 (-859.4753, -20) -> (-865.4753, -20)
  dimension "d37" = 6
  dimension "d38" = 6
  dimension "d39" = 6
  dimension "d40" = 6
  dimension "d42" = 30
  dimension "d43" = 30
  dimension "d44" = 50
  dimension "d47" = -870
  dimension "d48" = 0
  dimension "d49" = 50
  dimension "d52" = -870
  dimension "d53" = 0
  dimension "d54" = 30
  dimension "d55" = 30
  dimension "d56" = 50
  dimension "d59" = 0
  dimension "d60" = -270
  dimension "d61" = 50
  dimension "d64" = 0
  dimension "d65" = -270
  constraint coincident L21 L22.start
  constraint coincident L19 L22.end
  constraint perpendicular L19 L22
  constraint coincident L18 L23.start
  constraint coincident L20 L23.end
  constraint perpendicular L20 L23
  constraint coincident L21 L24.start
  constraint coincident L19 L24.end
  constraint perpendicular L19 L24
  constraint coincident L18 L25.start
  constraint coincident L20 L25.end
  constraint perpendicular L20 L25
  constraint coincident L22 L26.start
  constraint coincident L18 L26.end
  constraint perpendicular L18 L26
  constraint coincident L22 L27.start
  constraint coincident L18 L27.end
  constraint perpendicular L18 L27
  constraint horizontal L28
  constraint vertical L29
  constraint horizontal L30
  constraint vertical L31
  constraint coincident L18 L29.end
  constraint perpendicular L28 L68
  constraint perpendicular L20 L69
  constraint horizontal L70
  constraint vertical L71
  constraint horizontal L72
  constraint vertical L73
  constraint coincident L20 L71.end
  constraint coincident L68 L70.start
  constraint coincident L24 L70.start
  constraint perpendicular L25 L110
  constraint perpendicular L103 L111
  constraint horizontal L112
  constraint vertical L113
  constraint horizontal L114
  constraint vertical L115
  constraint coincident L21 L113.end
  constraint coincident L110 L112.start
  constraint coincident L23 L112.start
  constraint horizontal L128
  constraint vertical L129
  constraint horizontal L130
  constraint vertical L131
  constraint coincident L25 L129.end
  constraint coincident L19 L128.start
  constraint coincident L110 L128.start
  measures "d37" distance of L21 L23
  measures "d38" distance of L20 L24
  measures "d39" distance of L19 L25
  measures "d40" distance of L18 L22
  measures "d42" distance of L21 L26
  measures "d43" distance of L19 L27
  measures "d44" distance of L26.start L28.end
  measures "d49" distance of L70.start L70.end
  measures "d54" distance of L20 L111
  measures "d55" distance of L18 L110
  measures "d56" distance of L112.start L114.end
  measures "d61" distance of L128.start L130.end
extrude "Extrude2" cut sketch "Sketch2" against normal blind 40 contours L18 L28 L29 L30 L31 | L21 L112 L113 L114 L115 | L18 L32 L33 L34 L35 | L21 L116 L117 L118 L119 | L18 L36 L37 L38 L39 | L21 L120 L121 L122 L123 | L18 L40 L41 L42 L43 | L21 L124 L125 L126 L127 | L18 L44 L45 L46 L47 | L20 L70 L71 L72 L73 | L18 L48 L49 L50 L51 | L20 L74 L75 L76 L77 | L18 L52 L53 L54 L55 | L20 L78 L79 L80 L81 | L18 L56 L57 L58 L59 | L20 L82 L83 L84 L85 | L18 L60 L61 L62 L63 | L20 L86 L87 L88 L89 | L18 L27 L64 L65 L66 L67 | L20 L90 L91 L92 L93 | L19 L128 L129 L130 L131 | L20 L94 L95 L96 L97 | L19 L132 L133 L134 L135 | L20 L98 L99 L100 L101 | L19 L136 L137 L138 L139 | L20 L102 L103 L104 L105 | L19 L140 L141 L142 L143 | L20 L106 L107 L108 L109
equation "d7 = d6"
equation "d8 = d6"
equation "d10 = d6"
equation "d12 = d6"
equation "d23 = d22"
equation "d24 = d6"
equation "d28 = d22"
equation "d29 = d22"
equation "d30 = d6"
equation "d31 = d6"
equation "d32 = d6"
equation "d33 = d6"
